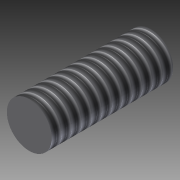
# Autodesk Inventor part: Small Gear Threaded Rod
Saved by Autodesk Inventor 2014 SP1 (Build 180222100, 222)
## iProperties
Created: 2012-03-30
Part Number: Small Gear Threaded Rod
Material: Generic
Document SubType Name: Modeling
Designer: Moses
Mass: 0.220244 g
Surface Area: 2.22166 cm^2
Volume: 0.220244 cm^3
Density: 1 g/cm^3
Appearance: Default
Author: Moses
Autodesk Inventor part; units mm, degrees
ref_plane "YZ Plane" through (0, 0, 0) normal (1, 0, 0) x (0, 1, 0)
ref_plane "XZ Plane" through (0, 0, 0) normal (0, 1, 0) x (-1, 0, 0)
ref_plane "XY Plane" through (0, 0, 0) normal (0, 0, 1) x (1, 0, 0)
sketch "Sketch1" plane through (0, 0, 0) normal (0, 0, 1) x (1, 0, 0)
  circle A0 centre (0, 0) radius 2.3495
  dimension "d0" = 4.699
  constraints: 1 centre point, 1 coincident
  measures "d0" diameter of A0
extrude "Extrusion1" add sketch "Sketch1" along normal blind 12.7
thread "Thread1" size "10-24 UNC" class "2A" standard "ANSI Unified Screw Threads" full length
body "Solid1"
